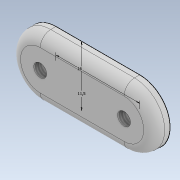
# Autodesk Inventor part: Connector_TopPlate
Saved by Autodesk Inventor 2022 (Build 260153000, 153)
## iProperties
Created: 2022-09-06
Part Number: Connector_TopPlate
Material: Generisch
Document SubType Name: Modeling
Designer: alexw
Density: 1 g/cm^3
Appearance: Vorgabe
Author: alexw
Autodesk Inventor part; units mm, degrees
ref_plane "YZ Plane" through (0, 0, 0) normal (1, 0, 0) x (0, 1, 0)
ref_plane "XZ Plane" through (0, 0, 0) normal (0, 1, 0) x (-1, 0, 0)
ref_plane "XY Plane" through (0, 0, 0) normal (0, 0, 1) x (1, 0, 0)
sketch "Skizze1" plane through (0, 0, 0) normal (0, 0, 1) x (1, 0, 0)
  line L0 (0, 0) -> (16, 0) construction
  line L1 (0, -5.75) -> (16, -5.75)
  line L2 (16, 5.75) -> (0, 5.75)
  arc A0 (0, 5.75) -> (0, -5.75) centre (0, 0) ccw
  arc A1 (16, -5.75) -> (16, 5.75) centre (16, 0) ccw
  point P0 (8, 0)
  dimension "d0" = 16
  dimension "d1" = 11.5
  constraints: 8 end point, 4 point on circle, 4 tangent, 2 centre point, 2 coincident, 1 horizontal, 1 midpoint, 1 parallel
  measures "d0" distance of L0.start L0.end
  measures "d1" distance between parallel lines of L1 L2
extrude "Extrusion1" add sketch "Skizze1" along normal blind 3
hole "Bohrung1" at (0, 0, 0) at (16, 0, 0) direction (0, 0, 1) diameter 2.459 end through all thread size "M3x0.5" class "6H" standard "ISO Metric profile"
fillet "Rundung1" radius 2 4 edges at (-5.75, 0, 3) (8, -5.75, 3) (21.75, 0, 3) (8, 5.75, 3)
